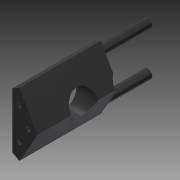
# Autodesk Inventor part: Support
Saved by Autodesk Inventor 2015 (Build 190159000, 159)
## iProperties
Created: 2015-11-27
Part Number: Support
Material: ABS Plastic
Document SubType Name: Modeling
Designer: James
Density: 1.06 g/cm^3
Appearance: Smooth - White
Mass: 16.1602 g
Surface Area: 69.4088 cm^2
Volume: 15.2455 cm^3
Author: James
Autodesk Inventor part; units mm, degrees
ref_plane "YZ Plane" through (0, 0, 0) normal (1, 0, 0) x (0, 1, 0)
ref_plane "XZ Plane" through (0, 0, 0) normal (0, 1, 0) x (-1, 0, 0)
ref_plane "XY Plane" through (0, 0, 0) normal (0, 0, 1) x (1, 0, 0)
sketch "Sketch1" plane through (0, 0, 0) normal (0, 1, 0) x (-1, 0, 0)
  line L0 (15.5801, 16.9856) -> (11.25, 19.4856)
  line L1 (11.25, -19.4856) -> (15.5801, -16.9856)
  line L2 (11.25, 19.4856) -> (0, 0)
  line L3 (0, 0) -> (11.25, -19.4856)
  line L4 (15.5801, 16.9856) -> (15.5801, -16.9856)
  circle A0 centre (5.625, 0) radius 1.4
  circle A1 centre (11.25, -9.7428) radius 1.4
  circle A2 centre (11.25, 9.7428) radius 1.4
  dimension "d4" = 2.8
  dimension "d5" = 2.8
  dimension "d6" = 2.8
  constraints: 10 end point, 3 centre point, 1 vertical
  measures "d4" diameter of A0
  measures "d5" diameter of A1
  measures "d6" diameter of A2
extrude "Extrusion1" add sketch "Sketch1" along normal blind 50
sketch "Sketch3" plane through (0, 50, 0) normal (0, 1, 0) x (1, 0, 0)
  circle A0 centre (-11.25, -9.7428) radius 1.4 projected
  circle A1 centre (-11.25, 9.7428) radius 1.4 projected
  circle A2 centre (-5.625, 0) radius 1.4 projected
  line L0 (-15.5801, -16.9856) -> (-11.25, -19.4856) projected
  line L1 (-11.25, -19.4856) -> (0, 0) projected
  line L2 (0, 0) -> (-11.25, 19.4856) projected
  line L3 (-11.25, 19.4856) -> (-15.5801, 16.9856) projected
  line L4 (-15.5801, 16.9856) -> (-15.5801, -16.9856) projected
  line L5 (-11.25, 0) -> (-15.5801, 16.9856)
  line L6 (-11.25, 0) -> (-15.5801, -16.9856)
  dimension "d15" = 5.625
  constraints: 4 end point
  measures "d15" distance of A2.centre L5.start
extrude "Extrusion3" add sketch "Sketch3" against normal blind 40 contours A0 | A1 | A2 | L4 L5 L6
sketch "Sketch4" plane through (0, 50, 0) normal (0, 1, 0) x (1, 0, 0)
  line L0 (-11.25, -19.4856) -> (-5.25, -19.4856) construction
  circle A0 centre (-12.2919, -13.5767) radius 1.4
  line L1 (0, 0) -> (-15.5801, 0)
  line L2 (-15.5801, 16.9856) -> (-15.5801, -16.9856) projected
  circle A1 centre (-12.2919, 13.5767) radius 1.4
  circle A2 centre (-12.2919, 13.5767) radius 2.75
  circle A3 centre (-12.2919, -13.5767) radius 2.75
  point P0 (-11.25, 19.4856)
  dimension "d12" = 2.8
  dimension "d78" = 5.5
  dimension "d79" = 5.5
  constraints: 4 centre point, 4 coincident, 4 end point, 2 symmetric about line, 1 horizontal, 1 midpoint, 1 other
  measures "d12" diameter of A0
  measures "d78" diameter of A2
  measures "d79" diameter of A3
extrude "Extrusion4" add sketch "Sketch4" along normal blind 30
sketch "Sketch6" plane through (-15.5801, 0, -16.9856) normal (-1, 0, 0) x (0, 0, 1)
  line L0 (16.9856, 15) -> (16.9856, 20)
  line L1 (16.9856, 50) -> (16.9856, 23) projected
  line L2 (16.9856, 20) -> (6.9856, 20)
  line L3 (26.9856, 20) -> (16.9856, 20)
  line L4 (6.9856, 20) -> (8.4856, 20)
  line L5 (8.4856, 20) -> (8.4856, 21.5)
  line L6 (26.9856, 20) -> (25.4856, 20)
  line L7 (25.4856, 20) -> (25.4856, 21.5)
  circle A0 centre (25.4856, 21.5) radius 0.6
  circle A1 centre (8.4856, 21.5) radius 0.6
  line L8 (16.9856, 20) -> (16.9856, 29)
  circle A2 centre (16.9856, 29) radius 8.5
  line L9 (16.9856, 29) -> (16.9856, 56)
  circle A3 centre (16.9856, 56) radius 8.5
  line L10 (26.9856, 20) -> (26.9856, 65)
  line L11 (26.9856, 65) -> (6.9856, 65)
  line L12 (6.9856, 65) -> (6.9856, 20)
  point P0 (16.9856, 0)
  dimension "d23" = 5
  dimension "d24" = 10
  dimension "d28" = 1.5
  dimension "d29" = 1.5
  dimension "d30" = 1.5
  dimension "d31" = 1.5
  dimension "d32" = 1.2
  dimension "d33" = 1.2
  dimension "d34" = 9
  dimension "d35" = 17
  dimension "d36" = 27
  dimension "d37" = 17
  dimension "d38" = 45
  dimension "d39" = 20
  constraints: 24 end point, 5 point on line, 4 centre point, 4 coincident, 3 perpendicular, 3 vertical, 2 horizontal
  measures "d23" distance of L0.start L0.end
  measures "d24" distance of L0.end L2.end
  measures "d28" distance of L2.end L4.end
  measures "d29" distance of L4.end L5.end
  measures "d30" distance of L3.start L6.end
  measures "d31" distance of L6.end L7.end
  measures "d32" diameter of A0
  measures "d33" diameter of A1
  measures "d34" distance of L0.end L8.end
  measures "d35" diameter of A2
  measures "d36" distance of L9.start L9.end
  measures "d37" diameter of A3
  measures "d38" distance of L3.start L10.end
  measures "d39" distance of L10.end L11.end
extrude "Extrusion6" cut sketch "Sketch6" against normal through all contours L1 A2 L8 | L1 L8 A2 | A3
sketch "Sketch7" plane through (-15.5801, 0, -16.9856) normal (-1, 0, 0) x (0, 0, 1)
  line L0 (16.9856, 15) -> (16.9856, 20)
  line L1 (16.9856, 50) -> (16.9856, 15)
  line L2 (16.9856, 20) -> (6.9856, 20)
  line L3 (26.9856, 20) -> (16.9856, 20)
  line L4 (6.9856, 20) -> (8.4856, 20)
  line L5 (8.4856, 20) -> (8.4856, 21.5)
  line L6 (26.9856, 20) -> (25.4856, 20)
  line L7 (25.4856, 20) -> (25.4856, 21.5)
  circle A0 centre (25.4856, 21.5) radius 0.9
  circle A1 centre (8.4856, 21.5) radius 0.9
  line L8 (16.9856, 20) -> (16.9856, 29)
  circle A2 centre (16.9856, 29) radius 8.5
  line L9 (16.9856, 29) -> (16.9856, 56)
  circle A3 centre (16.9856, 56) radius 8.5
  line L10 (26.9856, 20) -> (26.9856, 65)
  line L11 (26.9856, 65) -> (6.9856, 65)
  line L12 (6.9856, 65) -> (6.9856, 20)
  point P0 (16.9856, 0)
  point P1 (16.9856, 0)
  dimension "d42" = 5
  dimension "d43" = 10
  dimension "d44" = 1.5
  dimension "d45" = 1.5
  dimension "d46" = 1.5
  dimension "d47" = 1.5
  dimension "d48" = 1.8
  dimension "d49" = 1.8
  dimension "d50" = 9
  dimension "d51" = 17
  dimension "d52" = 27
  dimension "d53" = 17
  dimension "d54" = 45
  dimension "d55" = 20
  constraints: 26 end point, 5 point on line, 4 centre point, 4 coincident, 3 perpendicular, 3 vertical, 2 horizontal
  measures "d42" distance of L0.start L2.start
  measures "d43" distance of L2.start L2.end
  measures "d44" distance of L2.end L5.start
  measures "d45" distance of L5.start L5.end
  measures "d46" distance of L6.start L6.end
  measures "d47" distance of L6.end L7.end
  measures "d48" diameter of A0
  measures "d49" diameter of A1
  measures "d50" distance of L2.start L8.end
  measures "d51" diameter of A2
  measures "d52" distance of L9.start L9.end
  measures "d53" diameter of A3
  measures "d54" distance of L6.start L10.end
  measures "d55" distance of L10.end L12.start
extrude "Extrusion7" cut sketch "Sketch7" against normal blind 9 contours A0 | A1
sketch "Sketch8" plane through (-15.5801, 0, -16.9856) normal (-1, 0, 0) x (0, 0, 1)
  line L0 (5.9856, 20) -> (5.9856, 19)
  line L1 (28.0623, 50) -> (28.0623, 80) projected
  line L2 (26.9856, 66) -> (27.9856, 66)
  line L3 (27.9856, 66) -> (5.9856, 66)
  line L4 (5.9856, 66) -> (5.9856, 19)
  line L5 (5.9856, 19) -> (27.9856, 19)
  line L6 (27.9856, 19) -> (27.9856, 66)
  point P0 (16.9856, 0)
  point P1 (16.9856, 15)
  dimension "d73" = 1
  dimension "d75" = 1
  constraints: 12 end point, 2 parallel, 2 perpendicular, 1 horizontal
  measures "d73" distance of L0.start L0.end
  measures "d75" distance of L2.start L2.end
extrude "Extrusion8" cut sketch "Sketch8" against normal blind 2
body "Solid1"
